M3x3.8_94180A331_Tapered v1 (Autodesk Fusion 360 design; units mm, degrees)
Autodesk Fusion 360 part; units mm, degrees
sketch "Sketch1" plane through (0, 0, 0) normal (1, 0, 0) x (0, 1, 0)
  line L0 (0, 0) -> (0, 6.3486)
  line L1 (0, 6.3486) -> (2.98, 6.3486)
  line L2 (2.98, 6.3486) -> (2.98, 5.3486)
  line L3 (2.98, 5.3486) -> (2.6273, 4.9959)
  line L4 (2.6273, 4.9959) -> (2.6273, 1.5786)
  line L5 (2.6273, 1.5786) -> (0, 0)
  dimension "d1" = 59
  dimension "d2" = 5.2546
  dimension "d3" = 45
  dimension "d4" = 1
  dimension "d5" = 5.96
  dimension "d6" = 4.77
  constraint coincident L0.start L5.end
  constraint vertical L0
  constraint perpendicular L0 L1
  constraint perpendicular L1 L2
  constraint parallel L2 L4
  measures "d1" angle of L0 L5
  measures "d3" angle of L3 L4
  measures "d4" distance of L1 L2.end
  measures "d6" distance of L1 L4.end
revolve "Revolve1" add sketch "Sketch1" angle 360 about axis through (0, 0, 0) along (0, 0, 1)
equation "d1 = ( 118 / 2 ) * 1 deg"
equation "d2 = ( 0.199 * 25.4 ) * 1 mm + 0.2 mm"
equation "d5 = 5.56 mm + 0.4 mm"
equation "d6 = 4.57 mm + 0.2 mm"
